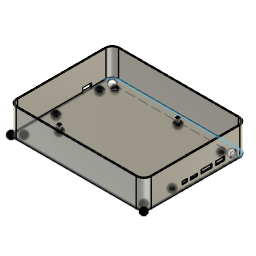
Mini PC Case V5 (Autodesk Fusion 360 design; units mm, degrees)
Autodesk Fusion 360 part; units mm, degrees
sketch "Sketch1" plane through (0, 0, 0) normal (0, 0, 1) x (1, 0, 0)
  line L0 (10, 0) -> (200, 0)
  line L1 (210, 10) -> (210, 150)
  line L2 (210, 150) -> (0, 150) construction
  line L3 (0, 150) -> (0, 10)
  circle A0 centre (118, 146) radius 1.65
  circle A1 centre (190, 143) radius 1.65
  line L4 (-2, 152) -> (-2, 10)
  line L5 (10, -2) -> (200, -2)
  line L6 (212, 10) -> (212, 152)
  circle A2 centre (201, 54) radius 1.65
  circle A3 centre (33.7, 42.5) radius 1.65
  line L7 (210, 143.8) -> (212, 143.8)
  line L8 (210, 135.5) -> (212, 135.5)
  line L9 (210, 126) -> (212, 126)
  line L10 (210, 112) -> (212, 112)
  line L11 (210, 106) -> (212, 106)
  line L12 (210, 89) -> (212, 89)
  line L13 (210, 83) -> (212, 83)
  line L14 (210, 72) -> (212, 72)
  line L15 (210, 67) -> (212, 67)
  line L16 (210, 59) -> (212, 59)
  circle A4 centre (33.7, 42.5) radius 2.5
  circle A5 centre (201, 54) radius 2.5
  circle A6 centre (190, 143) radius 2.5
  circle A7 centre (118, 146) radius 2.5
  circle A8 centre (10, 130) radius 1.65
  circle A9 centre (8.7, 62) radius 1.65
  circle A10 centre (10, 130) radius 2.5
  circle A11 centre (8.7, 62) radius 2.5
  line L17 (0, 127) -> (-2, 127)
  line L18 (-2, 113.5) -> (0, 113.5)
  circle A12 centre (20, 144.2) radius 4
  line L19 (212, 152) -> (212, 150)
  line L20 (200, 162) -> (10, 162)
  line L21 (-2, 150) -> (-2, 152)
  line L22 (210, 152) -> (210, 150)
  line L23 (200, 160) -> (10, 160)
  line L24 (0, 150) -> (0, 152)
  line L25 (210, 150) -> (210, 152)
  line L26 (0, 150) -> (0, 152)
  arc A13 (200, 0) -> (210, 10) centre (200, 10) ccw
  arc A14 (210, 150) -> (200, 160) centre (200, 150) ccw
  arc A15 (10, 160) -> (0, 150) centre (10, 150) ccw
  arc A16 (0, 10) -> (10, 0) centre (10, 10) ccw
  arc A17 (-2, 10) -> (10, -2) centre (10, 10) ccw
  arc A18 (200, -2) -> (212, 10) centre (200, 10) ccw
  arc A19 (212, 150) -> (200, 162) centre (200, 150) ccw
  arc A20 (10, 162) -> (-2, 150) centre (10, 150) ccw
  point P0 (210, 0)
  dimension "d1" = 210
  dimension "d2" = 150
  dimension "d8" = 3.3
  dimension "d9" = 3.3
  dimension "d24" = 3.3
  dimension "d29" = 3.3
  dimension "d31" = 107.5
  dimension "d33" = 6.2
  dimension "d34" = 14.5
  dimension "d35" = 24
  dimension "d36" = 38
  dimension "d37" = 44
  dimension "d38" = 61
  dimension "d39" = 67
  dimension "d40" = 78
  dimension "d41" = 83
  dimension "d42" = 91
  dimension "d46" = 5
  dimension "d48" = 5
  dimension "d49" = 5
  dimension "d50" = 5
  dimension "d53" = 3.3
  dimension "d54" = 20
  dimension "d55" = 10
  dimension "d56" = 3.3
  dimension "d57" = 88
  dimension "d58" = 8.7
  dimension "d59" = 5
  dimension "d60" = 5
  dimension "d65" = 23
  dimension "d66" = 36.5
  dimension "d67" = 8
  dimension "d68" = 20
  dimension "d69" = 5.8
  dimension "d80" = 10
  dimension "d81" = 12
  dimension "d102" = 9
  dimension "d103" = 96
  dimension "d104" = 20
  dimension "d105" = 7
  dimension "d107" = 4
  dimension "d108" = 92
  dimension "d109" = 176.3
  constraint horizontal L0
  constraint vertical L1
  constraint horizontal L2
  constraint vertical L3
  constraint coincident L1 L7.start
  constraint coincident L6 L7.end
  constraint perpendicular L6 L7
  constraint coincident L1 L8.start
  constraint coincident L6 L8.end
  constraint perpendicular L6 L8
  constraint coincident L1 L9.start
  constraint coincident L6 L9.end
  constraint perpendicular L6 L9
  constraint coincident L1 L10.start
  constraint coincident L6 L10.end
  constraint perpendicular L6 L10
  constraint coincident L1 L11.start
  constraint coincident L6 L11.end
  constraint perpendicular L6 L11
  constraint coincident L1 L12.start
  constraint coincident L6 L12.end
  constraint perpendicular L6 L12
  constraint coincident L1 L13.start
  constraint coincident L6 L13.end
  constraint perpendicular L6 L13
  constraint coincident L1 L14.start
  constraint coincident L6 L14.end
  constraint perpendicular L6 L14
  constraint coincident L1 L15.start
  constraint coincident L6 L15.end
  constraint perpendicular L6 L15
  constraint coincident L1 L16.start
  constraint coincident L6 L16.end
  constraint perpendicular L6 L16
  constraint concentric A3 A4
  constraint concentric A2 A5
  constraint concentric A1 A6
  constraint concentric A0 A7
  constraint concentric A8 A10
  constraint concentric A9 A11
  constraint coincident L3 L17.start
  constraint coincident L4 L17.end
  constraint perpendicular L4 L17
  constraint coincident L4 L18.start
  constraint coincident L3 L18.end
  constraint perpendicular L3 L18
  constraint perpendicular L4 L20
  constraint perpendicular L3 L23
  constraint coincident P0 L0
  constraint coincident P0 L1
  constraint tangent L0 A13
  constraint tangent L1 A13
  constraint tangent L22 A14
  constraint tangent L23 A14
  constraint equal A13 A14
  constraint tangent L23 A15
  constraint tangent L24 A15
  constraint equal A13 A15
  constraint coincident origin L0
  constraint coincident origin L3
  constraint tangent L0 A16
  constraint tangent L3 A16
  constraint equal A13 A16
  constraint tangent L4 A17
  constraint tangent L5 A17
  constraint tangent L5 A18
  constraint tangent L6 A18
  constraint equal A17 A18
  constraint tangent L19 A19
  constraint tangent L20 A19
  constraint equal A17 A19
  constraint tangent L20 A20
  constraint tangent L21 A20
  constraint equal A17 A20
  measures "d1" distance of origin P0
  measures "d2" distance of origin L2.end
  measures "d8" diameter of A0
  measures "d9" diameter of A1
  measures "d24" diameter of A2
  measures "d29" diameter of A3
  measures "d31" distance of L2 A3.centre
  measures "d33" distance of L1.end L7
  measures "d34" distance of L1.end L8
  measures "d35" distance of L1.end L9
  measures "d36" distance of L1.end L10
  measures "d37" distance of L1.end L11
  measures "d38" distance of L1.end L12
  measures "d39" distance of L1.end L13
  measures "d40" distance of L1.end L14
  measures "d41" distance of L1.end L15
  measures "d42" distance of L1.end L16
  measures "d46" diameter of A4
  measures "d48" diameter of A5
  measures "d49" diameter of A6
  measures "d50" diameter of A7
  measures "d53" diameter of A8
  measures "d54" distance of L2 A8.centre
  measures "d55" distance of L3 A8.centre
  measures "d56" diameter of A9
  measures "d57" distance of L2 A9.centre
  measures "d58" distance of L3 A9.centre
  measures "d59" diameter of A10
  measures "d60" diameter of A11
  measures "d65" distance of L2 L17
  measures "d66" distance of L2 L18
  measures "d67" diameter of A12
  measures "d68" distance of L3 A12.centre
  measures "d69" distance of L2 A12.centre
  measures "d80" radius of A13
  measures "d81" radius of A17
  measures "d102" distance of L1 A2.centre
  measures "d103" distance of L2 A2.centre
  measures "d104" distance of L1 A1.centre
  measures "d105" distance of L2 A1.centre
  measures "d107" distance of L2 A0.centre
  measures "d108" distance of L1 A0.centre
  measures "d109" distance of L1 A3.centre
extrude "Extrude1" add sketch "Sketch1" along normal blind 2 contours L0 L1 L3 L23 A13 A14 A15 A16 | L0 L1 L3 L4 L5 L6 L16 L18 A13 A16 A17 A18 | L3 L4 L17 L18 | L1 L6 L15 L16 | L1 L3 L4 L6 L7 L17 L20 L23 A14 A15 A19 A20 | L1 L6 L14 L15 | L1 L6 L13 L14 | L1 L6 L12 L13 | L1 L6 L11 L12 | L1 L6 L10 L11 | L1 L6 L7 L8 | L1 L6 L9 L10 | L1 L6 L8 L9 | A0 | A1 | A2 | A3 | A4 | A5 | A6 | A7 | A8 | A9 | A10 | A11
extrude "Extrude2" add sketch "Sketch1" along normal blind 44 contours L0 L1 L3 L4 L5 L6 L16 L18 A13 A16 A17 A18 | L1 L3 L4 L6 L7 L17 L20 L23 A14 A15 A19 A20 | L1 L6 L14 L15 | L1 L6 L12 L13 | L1 L6 L10 L11 | L1 L6 L8 L9
extrude "Extrude3" add sketch "Sketch1" along normal blind 10 contours A4 | A5 | A6 | A7
extrude "Extrude4" add sketch "Sketch1" along normal blind 5 contours A10 | A11
extrude "Extrude8" add sketch "Sketch1" along normal blind 44 and the other way blind -8 contours L3 L4 L17 L18
extrude "Extrude9" add sketch "Sketch1" along normal blind 7 contours L1 L6 L7 L8
extrude "Extrude10" add sketch "Sketch1" along normal blind 8 contours L1 L6 L15 L16 | L1 L6 L13 L14 | L1 L6 L11 L12 | L1 L6 L9 L10
extrude "Extrude11" add sketch "Sketch1" along normal blind 14 and the other way blind -44 contours L1 L6 L11 L12 | L1 L6 L7 L8 | L1 L6 L9 L10
extrude "Extrude12" add 1 faces at (210.6667, 79.3333, 8) along direction (0, 0, 1) blind 36 and the other way blind -4
extrude "Extrude13" add 1 faces at (210.6667, 64.3333, 8) along direction (0, 0, 1) blind 36 and the other way blind -5
equation "d8 = HolesRadius"
equation "d9 = HolesRadius"
equation "d24 = HolesRadius"
equation "d29 = HolesRadius"
equation "HolesRadius = 3.3 mm"
equation "d46 = HolesOuterRadius"
equation "HolesOuterRadius = 5 mm"
equation "d48 = HolesOuterRadius"
equation "d49 = HolesOuterRadius"
equation "d50 = HolesOuterRadius"
equation "d53 = HolesRadius"
equation "d56 = HolesRadius"
equation "d59 = HolesOuterRadius"
equation "d60 = HolesOuterRadius"
